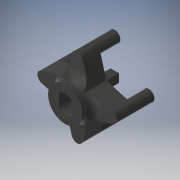
# Autodesk Inventor part: Wheel Mount
Saved by Autodesk Inventor 2019 (Build 230136000, 136)
## iProperties
Created: 2018-02-26
Part Number: Wheel Mount
Material: Generic
Document SubType Name: Modeling
Designer: Ethan
Density: 1 g/cm^3
Appearance: Smooth - Black
Author: Ethan
Autodesk Inventor part; units mm, degrees
ref_plane "YZ Plane" through (0, 0, 0) normal (1, 0, 0) x (0, 1, 0)
ref_plane "XZ Plane" through (0, 0, 0) normal (0, 1, 0) x (-1, 0, 0)
ref_plane "XY Plane" through (0, 0, 0) normal (0, 0, 1) x (1, 0, 0)
sketch "Sketch1" plane through (0, 0, 0) normal (0, 0, 1) x (1, 0, 0)
  circle A0 centre (0, 0) radius 3.4925
  line L0 (0, 0) -> (2.4032, 0) construction
  line L1 (2.4032, 2.5342) -> (2.4032, -2.5342)
  line L2 (0, 3.4925) -> (0, -3.4925) construction
  circle A1 centre (0, 0) radius 0.75 construction
  circle A2 centre (0, 0) radius 6.35
  line L3 (0, 0) -> (-2.4032, 0) construction
  line L4 (-2.4032, 2.5342) -> (-2.4032, -2.5342)
  dimension "d0" = 6.985
  dimension "d1" = 2.4032
  dimension "d2" = 12.7
  dimension "d3" = 1.5
  constraints: 10 end point, 6 point on circle, 3 centre point, 3 coincident, 3 midpoint, 2 vertical, 1 horizontal, 1 perpendicular, 1 symmetric about line
  measures "d0" diameter of A0
  measures "d1" distance of L0.end L0.start
  measures "d2" diameter of A2
  measures "d3" diameter of A1
extrude "Extrusion1" add sketch "Sketch1" against normal blind 10.795 contours A0 L1 | L1 A0 L4 | L4 A0 | A2
sketch "Sketch2" plane through (0, 0, -10.795) normal (0, 0, -1) x (-1, 0, 0)
  circle A0 centre (0, 0) radius 4
  line L0 (0, 0) -> (12.7, 0) construction
  circle A1 centre (12.7, 0) radius 3.175 construction
  circle A2 centre (0, 0) radius 2.5
  circle A3 centre (12.7, 0) radius 2.05
  line L1 (-1.55, -1.55) -> (1.55, -1.55)
  line L2 (1.55, -1.55) -> (1.55, 1.55)
  line L3 (1.55, 1.55) -> (-1.55, 1.55)
  line L4 (-1.55, 1.55) -> (-1.55, -1.55)
  line L5 (-1.55, -1.55) -> (1.55, 1.55) construction
  line L6 (1.55, -1.55) -> (-1.55, 1.55) construction
  circle A4 centre (0, 0) radius 6.35 projected
  line L7 (0, 0) -> (4.4901, 4.4901) construction
  line L8 (0, 0) -> (4.4901, -4.4901) construction
  line L9 (4.4901, 4.4901) -> (13.2658, 1.9704)
  line L10 (13.2658, -1.9704) -> (4.4901, -4.4901)
  point P0 (5.9927, 2.1)
  point P1 (5.6993, -2.8)
  dimension "d6" = 8
  dimension "d7" = 12.7
  dimension "d8" = 6.35
  dimension "d9" = 5
  dimension "d10" = 4.1
  dimension "d15" = 3.1
  constraints: 22 end point, 6 point on circle, 4 centre point, 4 coincident, 3 perpendicular, 2 horizontal, 2 parallel, 2 tangent, 1 midpoint, 1 point on line, 1 other
  measures "d6" diameter of A0
  measures "d7" distance of L0.start L0.end
  measures "d8" diameter of A1
  measures "d9" diameter of A2
  measures "d10" diameter of A3
  measures "d15" distance of L3.end L2.end
extrude "Extrusion2" add sketch "Sketch2" against normal blind 6.35 contours A0 | A2 | A3 | A3 L10 A4 L9 | A4 | L4 L3 L2 L1
extrude "Extrusion3" add sketch "Sketch2" along normal blind 7.62 contours L4 L3 L2 L1
extrude "Extrusion4" add sketch "Sketch2" along normal blind 7.62 contours A3
pattern_circular "Circular Pattern1" count 4 over 360 about axis through (0, 0, -10) along (0, 0, 1) of "Extrusion2", "Extrusion4"
extrude "Extrusion5" cut sketch "Sketch1" against normal blind 6.35 contours L1 A0 L4
fillet "Fillet1" [suppressed]
fillet "Fillet2" radius 3.175 5 edges at (-6.35, 0, -4.445) (0, 6.35, -4.445) (5.8666, 2.43, -4.445) (5.8666, -2.43, -4.445) (0, -6.35, -4.445)
fillet "Fillet3" [suppressed]
feature "Move Body1" [suppressed]
equation "\"d32\" = d34"
equation "\"d34\" = 7.62"
body "Solid1"
